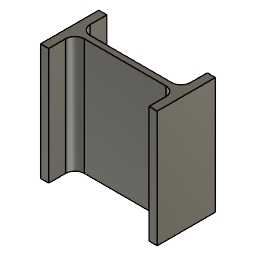
H-100×50×5×7 (Autodesk Fusion 360 design; units mm, degrees)
Autodesk Fusion 360 part; units mm, degrees
sketch "スケッチ1" plane through (0, 0, 0) normal (0, 0, 1) x (1, 0, 0)
  line L0 (0, 25) -> (0, -25)
  line L1 (100, -25) -> (100, 25)
  line L2 (93, -10.5) -> (93, -25)
  line L3 (7, -25) -> (7, -10.5)
  line L4 (0, -25) -> (7, -25)
  line L5 (93, -25) -> (100, -25)
  line L6 (85, 2.5) -> (15, 2.5)
  line L7 (15, -2.5) -> (85, -2.5)
  line L8 (7, 10.5) -> (7, 25)
  arc A0 (7, 10.5) -> (15, 2.5) centre (15, 10.5) ccw
  arc A1 (15, -2.5) -> (7, -10.5) centre (15, -10.5) ccw
  line L9 (7, 25) -> (0, 25)
  line L10 (93, 25) -> (93, 10.5)
  arc A2 (85, 2.5) -> (93, 10.5) centre (85, 10.5) ccw
  arc A3 (93, -10.5) -> (85, -2.5) centre (85, -10.5) ccw
  line L11 (100, 25) -> (93, 25)
extrude "押し出し1" add sketch "スケッチ1" along normal blind 100
